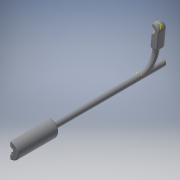
# Autodesk Inventor part: lampa
Saved by Autodesk Inventor 2018 (Build 220112000, 112)
## iProperties
Created: 2018-12-13
Part Number: lampa
Material: Generic
Document SubType Name: Modeling
Designer: petal
Density: 1 g/cm^3
Appearance: Default
Author: petal
Autodesk Inventor part; units mm, degrees
ref_plane "YZ Plane" through (0, 0, 0) normal (1, 0, 0) x (0, 1, 0)
ref_plane "XZ Plane" through (0, 0, 0) normal (0, 1, 0) x (-1, 0, 0)
ref_plane "XY Plane" through (0, 0, 0) normal (0, 0, 1) x (1, 0, 0)
sketch "Sketch1" plane through (0, 0, 0) normal (0, 0, 1) x (1, 0, 0)
  line L0 (0, 0) -> (0, 150)
  line L1 (0, 150) -> (3, 150) construction
  line L2 (3, 150) -> (3, 40)
  line L3 (0, 0) -> (8, 0)
  line L4 (8, 0) -> (8, 40)
  line L5 (8, 40) -> (3, 40)
  line L6 (1.844, 1) -> (3.3005, 1)
  line L7 (3.3005, 1) -> (3.3005, 0)
  line L8 (1.844, 1) -> (1.844, 2)
  line L9 (1.844, 2) -> (6.5, 2)
  line L10 (6.5, 2) -> (6.5, 38.5)
  line L11 (6.5, 38.5) -> (1.5, 38.5)
  line L12 (1.5, 38.5) -> (1.5, 148.1426)
  line L13 (1.5, 148.1426) -> (1.5, 150)
  line L14 (1.5, 149) -> (0.5, 149)
  line L15 (0.5, 149) -> (0.5, 148)
  line L16 (0.5, 148) -> (1.5, 148)
  line L17 (1.5, 150) -> (3, 150)
  dimension "d0" = 150
  dimension "d1" = 3
  dimension "d3" = 8
  dimension "d4" = 40
  dimension "d20" = 1.5
  dimension "d21" = 1.5
  dimension "d22" = 1.5
  dimension "d23" = 1
  dimension "d24" = 1
  dimension "d25" = 1
  dimension "d26" = 1
  dimension "d27" = 1
  dimension "d28" = 1.4566
  dimension "d29" = 6.601
  dimension "d51" = 3
  constraints: 36 end point, 9 perpendicular, 4 horizontal, 4 vertical, 3 point on line, 1 collinear, 1 midpoint
  measures "d0" distance of L0.start L0.end
  measures "d1" distance of L0.end L1.end
  measures "d3" distance of L0.start L3.end
  measures "d4" distance of L3.end L4.end
  measures "d20" distance between parallel lines of L4 L10
  measures "d21" distance between parallel lines of L2 L12
  measures "d22" distance between parallel lines of L5 L11
  measures "d23" distance of L15.end L14.end
  measures "d24" distance of L14.start L14.end
  measures "d25" distance of L13.end L14.start
  measures "d26" distance from line of L3.end L6
  measures "d27" distance of L8.end L6.start
  measures "d28" distance between parallel lines of L7 L8
  measures "d29" diameter of L7 L0
  measures "d51" diameter of L13 L0
revolve "Revolution1" add sketch "Sketch1" angle 360 about axis through (0, 0, 0) along (0, 1, 0)
fillet "Fillet1" radius 2 1 edges at (-8, 40, 0)
fillet "Fillet2" radius 1 1 edges at (-8, 0, 0)
fillet "Fillet3" radius 1 1 edges at (-3, 150, 0)
ref_plane "Work Plane1" through (0, 126, 0) normal (0, 1, 0) x (1, 0, 0)
sketch "Sketch6" plane through (0, 126, 0) normal (0, 1, 0) x (1, 0, 0)
  circle A0 centre (0, 0) radius 3 projected
  circle A1 centre (0, 0) radius 1.5 projected
sketch "Sketch8" plane through (0, 0, 0) normal (1, 0, 0) x (0, 1, 0)
  arc A0 (126, 0) -> (142, 18) centre (124.0003, 17.8886) ccw
  point P0 (0, 0)
  dimension "d38" = 18
  dimension "d39" = 18
  dimension "d40" = 16
  constraints: 2 point on circle, 1 centre point
  measures "d38" radius of A0
  measures "d39" vertical distance of A0.start A0.end
  measures "d40" horizontal distance of A0.start A0.end
sweep "Sweep1" add profiles "Sketch6" path "Sketch8"
sketch "Sketch9" plane through (0, 142, 18) normal (0, 0.1049383, 0.9944787) x (1, 0, 0)
  circle A0 centre (0, 0) radius 1.5 projected
  circle A1 centre (0, 0) radius 3 projected
  line L0 (-6, -5) -> (6, -5)
  arc A2 (6, 0) -> (-6, 0) centre (0, 0) ccw
  line L1 (6, -5) -> (6, 0)
  line L2 (-6, -5) -> (-6, 0)
  point P0 (0, -139.3271)
  point P1 (1.5, 0)
  point P2 (3, 0)
  dimension "d43" = 12
  dimension "d44" = 5
  dimension "d45" = 6
  dimension "d46" = 6
  constraints: 6 end point, 2 horizontal alignment, 2 point on circle, 2 tangent, 1 centre point, 1 coincident, 1 horizontal
  measures "d43" diameter of A2
  measures "d44" distance from line of L0 point (0, 0)
  measures "d45" horizontal distance of L0.end point (0, 0)
  measures "d46" horizontal distance of L0.start point (0, 0)
extrude "Extrusion2" add sketch "Sketch9" along normal blind 20 contours A0 | A1 | L2 A2 L1 L0
fillet "Fillet4" radius 6 3 edges at (-6, 141.6126, 38.1519) (6, 141.6126, 38.1519) (0, 150.0656, 37.2599)
fillet "Fillet5" radius 1 12 edges at (-6, 139.5138, 18.2623) (6, 139.5138, 18.2623) (0, 147.9669, 17.3704) (0, 139.0166, 18.3148) (0, 144.9834, 17.6852) (-0.0034, 138.7876, 3) (-4.2427, 138.942, 36.6666) (0, 139.1264, 38.4143) (4.2427, 138.942, 36.6666) (-6, 137.7622, 25.4861) (6, 137.7622, 25.4861) (0, 137.0276, 18.5247)
sketch "Sketch10" plane through (0, 138.4967, 32.4474) normal (0, -0.9944787, 0.1049383) x (1, 0, 0)
  line L0 (5, -13) -> (-5, -13) projected
  line L1 (5, 0) -> (5, -13) projected
  arc A0 (5, 0) -> (-5, 0) centre (0, 0) ccw projected
  line L2 (-5, -13) -> (-5, 0) projected
  circle A1 centre (0, 0) radius 2.75
  point P0 (0, -46.8019)
  dimension "d52" = 5.5
  constraints: 1 centre point, 1 coincident
  measures "d52" diameter of A1
extrude "Extrusion3" cut sketch "Sketch10" against normal blind 8 contours A1
sketch "Sketch11" plane through (0, 0, 0) normal (1, 0, 0) x (0, 1, 0)
  line L0 (163.7733, 50.4926) -> (0, 50.4926)
  line L1 (0, 50.4926) -> (0, -25.116)
  line L2 (0, -25.116) -> (163.7733, -25.116)
  line L3 (163.7733, -25.116) -> (163.7733, 50.4926)
  point P0 (0, 0)
  constraints: 8 end point, 2 parallel, 1 horizontal, 1 perpendicular
extrude "Extrusion4" cut sketch "Sketch11" against normal blind 10
sketch "Sketch12" plane through (0, 148, 0) normal (0, -1, 0) x (1, 0, 0)
  arc A0 (0, -1.5) -> (0, 1.5) centre (0, 0) ccw projected
  circle A1 centre (0, 0) radius 1.5
  constraints: 1 coincident, 1 vertical alignment, 2 other
extrude "Extrusion5" cut sketch "Sketch12" along normal blind 50
sketch "Sketch13" plane through (0, 0, 0) normal (-1, 0, 0) x (0, 0, 1)
  line L0 (1.5, 148) -> (1.5, 38.5) projected
  line L1 (3, 136.5799) -> (3, 131.1358) projected
  line L2 (3, 135.7743) -> (-0.254, 135.7743)
  line L3 (-0.254, 135.7743) -> (-0.254, 131.4421)
  line L4 (-0.254, 131.4421) -> (3, 131.4421)
  line L5 (3, 131.4421) -> (3, 135.7743)
  point P0 (0, 0)
  point P1 (1.5, 136.6682)
  point P2 (3, 132.1721)
  dimension "d61" = 4.3322
  constraints: 8 end point, 3 point on line, 2 parallel, 1 horizontal, 1 perpendicular
  measures "d61" distance of L2.end L3.end
extrude "Extrusion6" cut sketch "Sketch13" against normal blind 1.4
sketch "Sketch14" plane through (0, 142, 18) normal (0, -0.1049383, -0.9944787) x (-1, 0, 0)
  line L0 (0, -1.5) -> (0, 1.5) projected
  arc A0 (0, 1.5) -> (-1.5, 0) centre (0, 0) ccw projected
  circle A1 centre (0, 0) radius 1.5
  point P0 (0, -139.3271)
  constraints: 1 horizontal alignment, 1 midpoint, 2 other
extrude "Extrusion7" cut sketch "Sketch14" against normal blind 15
ref_plane "Work Plane3" through (0, 140.116, 19.2044) normal (0, -0.9944787, 0.1049383) x (1, 0, 0)
sketch "Sketch15" plane through (0, 140.116, 19.2044) normal (0, -0.9944787, 0.1049383) x (1, 0, 0)
  line L0 (0, 15.75) -> (0, 10.25) projected
  arc A0 (0, 10.25) -> (0, 15.75) centre (0, 13) ccw projected
  line L1 (6, 13) -> (0, 13) projected
  circle A1 centre (0, 13) radius 3.25
  point P0 (0, -33.8019)
  dimension "d65" = 6.5
  constraints: 1 centre point, 1 coincident
  measures "d65" diameter of A1
extrude "Extrusion8" cut sketch "Sketch15" along normal mid plane 1.1
equation "\"d46\" = d45"
equation "\"d21\" = d22"
equation "\"d22\" = d20"
body "Solid1"
